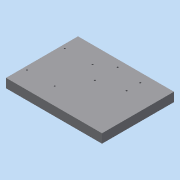
# Autodesk Inventor part: base of car
Saved by Autodesk Inventor 2015 (Build 190159000, 159)
## iProperties
Created: 2015-06-23
Part Number: base of car
Material: Generic
Document SubType Name: Modeling
Designer: Rahul
Density: 1 g/cm^3
Appearance: Default
Author: Rahul
Autodesk Inventor part; units mm, degrees
ref_plane "YZ Plane" through (0, 0, 0) normal (1, 0, 0) x (0, 1, 0)
ref_plane "XZ Plane" through (0, 0, 0) normal (0, 1, 0) x (-1, 0, 0)
ref_plane "XY Plane" through (0, 0, 0) normal (0, 0, 1) x (1, 0, 0)
sketch "Sketch1" plane through (0, 0, 0) normal (0, 0, 1) x (1, 0, 0)
  line L0 (-142.24, 0) -> (142.24, 0) projected
  line L1 (0, -106.68) -> (0, 106.68) projected
  line L2 (-101.6, -76.2) -> (101.6, -76.2)
  line L3 (101.6, -76.2) -> (101.6, 76.2)
  line L4 (101.6, 76.2) -> (-101.6, 76.2)
  line L5 (-101.6, 76.2) -> (-101.6, -76.2)
  point P0 (0, 0)
  dimension "d0" = 203.2
  dimension "d1" = 152.4
  constraints: 8 end point, 2 parallel, 1 perpendicular, 2 other
  measures "d0" distance of L2.start L2.end
  measures "d1" distance of L2.end L3.end
extrude "Extrusion1" add sketch "Sketch1" along normal blind 19.05
sketch "Sketch14" plane through (0, 0, 0) normal (0, 0, -1) x (-1, 0, 0)
  circle A0 centre (-49.4284, -56.9976) radius 1.7653
  line L0 (-101.6, -76.2) -> (-101.6, 76.2) projected
  circle A1 centre (-49.4284, -28.1432) radius 1.7653
  circle A2 centre (2.7686, -61.214) radius 1.7653
  line L1 (101.6, -76.2) -> (-101.6, -76.2) projected
  circle A3 centre (2.7686, -13.1826) radius 1.7653
  line L2 (101.6, 76.2) -> (101.6, -76.2) projected
  point P0 (0, 0)
  dimension "d20" = 3.5306
  dimension "d21" = 28.8544
  dimension "d22" = 3.5306
  dimension "d23" = 14.986
  dimension "d24" = 3.5306
  dimension "d26" = 63.0174
  dimension "d27" = 19.2024
  dimension "d28" = 3.5306
  dimension "d36" = 52.1716
  dimension "d37" = 52.1716
  dimension "d38" = 104.3686
  dimension "d39" = 104.3686
  constraints: 4 centre point
  measures "d20" diameter of A0
  measures "d21" distance of A1.centre A0.centre
  measures "d22" diameter of A1
  measures "d23" distance from line of A2.centre L1
  measures "d24" diameter of A2
  measures "d26" distance from line of L1 A3.centre
  measures "d27" distance from line of A0.centre L1
  measures "d28" diameter of A3
  measures "d36" distance from line of L0 A1.centre
  measures "d37" distance from line of L0 A0.centre
  measures "d38" distance from line of L0 A3.centre
  measures "d39" distance from line of L0 A2.centre
extrude "Extrusion7" cut sketch "Sketch14" against normal blind 25.4
sketch "Sketch17" plane through (0, 0, 0) normal (0, 0, -1) x (-1, 0, 0)
  circle A0 centre (34.3916, -39.8272) radius 1.5875
  line L0 (101.6, -76.2) -> (-101.6, -76.2) projected
  line L1 (101.6, 76.2) -> (101.6, -76.2) projected
  circle A1 centre (93.1418, -39.8272) radius 1.5875
  circle A2 centre (34.925, 39.5986) radius 1.5875
  circle A3 centre (93.6498, 39.5986) radius 1.5875
  line L2 (-101.6, 76.2) -> (101.6, 76.2) projected
  point P0 (0, 0)
  dimension "d48" = 36.3728
  dimension "d49" = 3.175
  dimension "d50" = 67.2084
  dimension "d51" = 8.4582
  dimension "d52" = 3.175
  dimension "d53" = 36.3728
  dimension "d54" = 66.675
  dimension "d55" = 3.175
  dimension "d56" = 7.9502
  dimension "d59" = 36.6014
  dimension "d60" = 36.6014
  constraints: 4 centre point
  measures "d48" distance from line of L0 A0.centre
  measures "d49" diameter of A0
  measures "d50" distance from line of L1 A0.centre
  measures "d51" distance from line of L1 A1.centre
  measures "d52" diameter of A1
  measures "d53" distance from line of L0 A1.centre
  measures "d54" distance from line of L1 A2.centre
  measures "d55" diameter of A2
  measures "d56" distance from line of L1 A3.centre
  measures "d59" distance from line of L2 A2.centre
  measures "d60" distance from line of L2 A3.centre
extrude "Extrusion9" cut sketch "Sketch17" against normal blind 19.05
body "Solid1"
